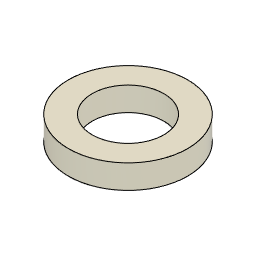
Volume Assembly v5 (Autodesk Fusion 360 archive; units mm, degrees)
design "Washer"
Autodesk Fusion 360 part; units mm, degrees
sketch "Sketch1" plane through (0, 0, 0) normal (0, 1, 0) x (1, 0, 0)
  circle A0 centre (0, 0) radius 5
  circle A1 centre (0, 0) radius 3
  dimension "d1" = 6
  dimension "d2" = 10
  constraint coincident A0.centre A1.centre
  constraint concentric A0 A1
  measures "d1" diameter of A1
  measures "d2" diameter of A0
extrude "Extrude1" add sketch "Sketch1" along normal blind 2

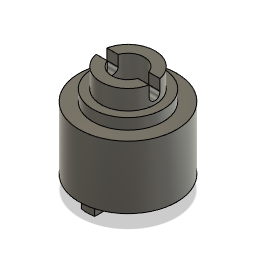
design "TOK_TLE1-618-5W"
Autodesk Fusion 360 part; units mm, degrees
sketch "Sketch1" plane through (0, 0, 0) normal (0, 0, 1) x (1, 0, 0)
  line L0 (0, 0) -> (0, 35)
  line L1 (3, 17.2) -> (3, 0)
  line L2 (3, 0) -> (9, 0)
  line L3 (9, 0) -> (9, 11.6)
  line L4 (9, 11.6) -> (6.5, 11.6)
  line L5 (6.5, 11.6) -> (6.5, 13.6)
  line L6 (6.5, 13.6) -> (5, 13.6)
  line L7 (5, 13.6) -> (5, 17.2)
  line L8 (5, 17.2) -> (3, 17.2)
  dimension "d1" = 6
  dimension "d2" = 18
  dimension "d3" = 11.6
  dimension "d4" = 13
  dimension "d5" = 10
  dimension "d6" = 2
  dimension "d7" = 17.2
  constraint coincident L0.start origin
  constraint vertical L0
  constraint parallel L0 L1
  constraint perpendicular L1 L2
  constraint perpendicular L2 L3
  constraint perpendicular L3 L4
  constraint perpendicular L4 L5
  constraint perpendicular L5 L6
  constraint perpendicular L6 L7
  constraint perpendicular L7 L8
  constraint coincident L0.start L2
  measures "d3" distance of L2.end L3.end
  measures "d6" distance of L4.end L5.end
  measures "d7" distance of L2 L8
revolve "Revolve1" add sketch "Sketch1" angle 360 about axis through (0, 0, 0) along (0, 1, 0)
sketch "Sketch2" plane through (0, 0, 0) normal (1, 0, 0) x (0, 0, -1)
  line L0 (-1, 17.2) -> (-1, 15.2)
  arc A0 (-1, 15.2) -> (1, 15.2) centre (0, 15.2) ccw
  line L1 (1, 15.2) -> (1, 17.2)
  arc A1 (1, 17.2) -> (-1, 17.2) centre (0, 17.2) ccw
  line L2 (0, 17.2) -> (0, 15.2) construction
  line L3 (-5, 17.2) -> (5, 17.2)
  dimension "d9" = 2
  dimension "d10" = 1
  constraint tangent L0 A0
  constraint tangent A0 L1
  constraint parallel L0 L1
  constraint tangent L1 A1
  constraint tangent L0 A1
  constraint vertical L2
  constraint coincident A1.centre L3
  constraint midpoint A1.centre L3
  measures "d9" distance of A1.centre A0.centre
  measures "d10" radius of A1
extrude "Extrude1" cut sketch "Sketch2" along normal through all and the other way through all contours L0 A0 L1 L3
sketch "Sketch3" plane through (0, 0, 0) normal (0, -1, 0) x (1, 0, 0)
  circle A0 centre (0, 0) radius 9
  circle A1 centre (0, 0) radius 3
  line L0 (-1.225, 5.3618) -> (-1.225, 7.3993)
  line L1 (1.225, 7.3993) -> (1.225, 5.3618)
  line L2 (1.225, 5.3618) -> (-1.225, 7.3993) construction
  line L3 (-1.225, 5.3618) -> (1.225, 7.3993) construction
  arc A2 (1.225, 5.3618) -> (-1.225, 5.3618) centre (0, 0) ccw
  arc A3 (1.225, 7.3993) -> (-1.225, 7.3993) centre (0, 0) ccw
  line L4 (0, 7.5) -> (0, 0) construction
  point P0 (0, 6.3806)
  dimension "d12" = 2.45
  dimension "d13" = 2
  dimension "d14" = 7.5
  constraint parallel L0 L1
  constraint coincident L2 P0
  constraint coincident L3 P0
  constraint coincident A0.centre A1.centre
  constraint midpoint A3 L4.start
  constraint vertical L4
  constraint vertical A0.centre P0
  measures "d12" distance of L0.end L1.start
  measures "d13" distance of A2 A3
  measures "d14" distance of L4.start A0.centre
extrude "Extrude2" add sketch "Sketch3" along normal blind 2.5 contours L0 L1 A2 A3
pattern_circular "C-Pattern1" count 2 over 360 about axis through (0, 17.2, 0) along (0, -1, 0) of "Extrude2"
equation "d14 = ( 15 / 2 ) * 1 mm"
